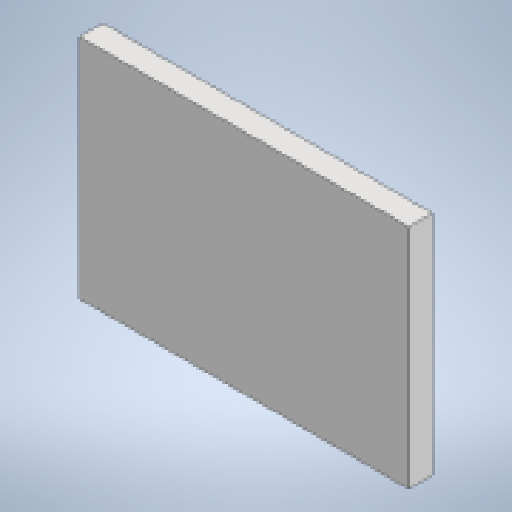
# Autodesk Inventor part: 부품74
Saved by Autodesk Inventor 2024 (Build 280153000, 153)
## iProperties
Created: 2024-09-08
Part Number: 부품74
Material: PMMA 플라스틱
Document SubType Name: Modeling
Designer: Eungang
Mass: 33.6002 g
Surface Area: 117.397 cm^2
Volume: 28.283 cm^3
Density: 1.188 g/cm^3
Appearance: 폴리카보네이트 - 선명
Author: Eungang
Autodesk Inventor part; units mm, degrees
ref_plane "YZ Plane" through (0, 0, 0) normal (1, 0, 0) x (0, 1, 0)
ref_plane "XZ Plane" through (0, 0, 0) normal (0, 1, 0) x (-1, 0, 0)
ref_plane "XY Plane" through (0, 0, 0) normal (0, 0, 1) x (1, 0, 0)
sketch "스케치1" plane through (0, 0, 0) normal (0, 0, 1) x (1, 0, 0)
  line L0 (-12.2, 0) -> (71.7, 0) projected
  line L1 (71.7, 5.8) -> (71.7, 0) projected
  line L2 (-12.2, 5.8) -> (71.7, 5.8) projected
  line L3 (-12.2, 5.8) -> (-12.2, 0) projected
  line L4 (-12.2, -46.0408) -> (71.7, -46.0408) projected
  line L5 (71.7, -40.2408) -> (71.7, -46.0408) projected
  line L6 (-12.2, -40.2408) -> (71.7, -40.2408) projected
  line L7 (-12.2, -40.2408) -> (-12.2, -46.0408) projected
  line L8 (-12.2, -46.0408) -> (71.7, -46.0408)
  line L9 (71.7, -46.0408) -> (71.7, 17.8002)
  line L10 (71.7, 17.8002) -> (-12.2, 17.8002)
  line L11 (-12.2, 17.8002) -> (-12.2, -46.0408)
  point P0 (0, 0)
  dimension "d0" = 63.841
  constraints: 8 end point, 2 parallel, 1 horizontal, 1 perpendicular
  measures "d0" distance of L9.end L8.end
extrude "돌출1" add sketch "스케치1" along normal blind 6
sketch "스케치2" plane through (0, 0, 6) normal (0, 0, 1) x (1, 0, 0)
  circle A0 centre (15, -19.9408) radius 14.3
  point P0 (0, 0)
  constraints: 1 centre point
extrude "돌출2" cut sketch "스케치2" against normal blind 6
